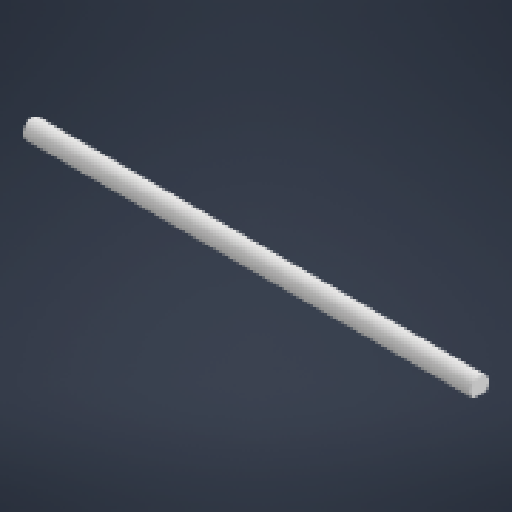
# Autodesk Inventor part: Axle3dprinted
Saved by Autodesk Inventor 2024.1 (Build 281209000, 209)
## iProperties
Created: 2023-10-19
Part Number: Axle3dprinted
Material: Generic
Document SubType Name: Modeling
Designer: Brandon
Density: 1 g/cm^3
Appearance: Default
Author: Brandon
Autodesk Inventor part; units mm, degrees
ref_plane "YZ Plane" through (0, 0, 0) normal (1, 0, 0) x (0, 1, 0)
ref_plane "XZ Plane" through (0, 0, 0) normal (0, 1, 0) x (-1, 0, 0)
ref_plane "XY Plane" through (0, 0, 0) normal (0, 0, 1) x (1, 0, 0)
sketch "Sketch1" plane through (0, 0, 0) normal (1, 0, 0) x (0, 1, 0)
  circle A0 centre (0, 0) radius 2.9845
  line L0 (-2.11036, 2.11036) -> (-2.11036, -2.11036)
  line L1 (-2.11036, -2.11036) -> (0.965216, -5.185936)
  line L2 (-2.11036, -2.11036) -> (2.239161, -2.11036) construction
  dimension "d0" = 5.969
  dimension "d1" = 45
  constraints: 6 end point, 2 point on circle, 1 centre point, 1 coincident, 1 equal length, 1 horizontal, 1 tangent, 1 vertical
  measures "d0" diameter of A0
  measures "d1" angle of L1 L2
sketch "Sketch1 outline for Extrusion1" plane through (0, 0, 0) normal (1, 0, 0) x (0, 1, 0)
  line L0 (-2.11036, 2.11036) -> (-2.11036, -2.11036)
  arc A0 (-2.11036, -2.11036) -> (-2.11036, 2.11036) centre (0, 0) ccw
extrude "Extrusion1" add sketch "Sketch1 outline for Extrusion1" along normal blind 150
chamfer "Chamfer1" distance 0.635 angle 45 2 edges at (0, 2.9845, 0) (150, 2.9845, 0)
body "Solid1"
